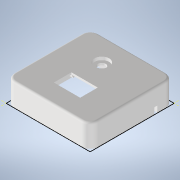
# Autodesk Inventor part: Deckel
Saved by Autodesk Inventor 2022.2 (Build 262287000, 287)
## iProperties
Created: 2022-01-23
Part Number: Deckel
Material: Generisch
Document SubType Name: Modeling
Designer: hpcwoess
Density: 1 g/cm^3
Appearance: Vorgabe
Author: hpcwoess
Autodesk Inventor part; units mm, degrees
ref_plane "YZ Plane" through (0, 0, 0) normal (1, 0, 0) x (0, 1, 0)
ref_plane "XZ Plane" through (0, 0, 0) normal (0, 1, 0) x (-1, 0, 0)
ref_plane "XY Plane" through (0, 0, 0) normal (0, 0, 1) x (1, 0, 0)
sketch "Skizze1" plane through (0, 0, 0) normal (0, 1, 0) x (-1, 0, 0)
  line L0 (30.3, 19.3) -> (-30.3, 19.3)
  line L1 (-30.3, 19.3) -> (-30.3, -34.9)
  line L2 (-30.3, -34.9) -> (30.3, -34.9)
  line L3 (30.3, -34.9) -> (30.3, 19.3)
  line L4 (40.5, -43.7) -> (-40.5, -43.7)
  line L5 (-40.5, -43.7) -> (-40.5, 37.3)
  line L6 (-40.5, 37.3) -> (40.5, 37.3)
  line L7 (40.5, 37.3) -> (40.5, -43.7)
  point P0 (0, 0)
  dimension "d0" = 30.3
  dimension "d1" = 60.6
  dimension "d2" = 54.2
  dimension "d3" = 19.3
  dimension "d4" = 81
  dimension "d5" = 81
  dimension "d6" = 40.5
  dimension "d7" = 18
  constraints: 16 end point, 4 parallel, 2 horizontal, 2 perpendicular
  measures "d0" distance from line of L3 point (0, 0)
  measures "d1" distance of L0.start L0.end
  measures "d2" distance of L2.end L0.start
  measures "d3" distance from line of L0 point (0, 0)
  measures "d4" distance of L5.end L6.end
  measures "d5" distance of L4.end L5.end
  measures "d6" distance from line of L5 point (0, 0)
  measures "d7" distance between parallel lines of L6 L0
extrude "Extrusion1" add sketch "Skizze1" along normal blind 20
sketch "Skizze2" plane through (0, 0, 0) normal (0, -1, 0) x (1, 0, 0)
  line L0 (-40.5, 37.3) -> (40.5, 37.3)
  line L1 (40.5, 37.3) -> (40.5, -43.7)
  line L2 (40.5, -43.7) -> (-40.5, -43.7)
  line L3 (-40.5, -43.7) -> (-40.5, 37.3)
  point P0 (0, 0)
  constraints: 8 end point, 2 parallel, 1 horizontal, 1 perpendicular
sketch "Skizze3" plane through (0, 20, 0) normal (0, 1, 0) x (1, 0, 0)
  line L0 (30.3, -19.3) -> (-30.3, -19.3) projected
  line L1 (25, -19.3) -> (-25, -19.3)
  line L2 (-25, -19.3) -> (-25, -31.3)
  line L3 (-25, -31.3) -> (25, -31.3)
  line L4 (25, -31.3) -> (25, -19.3)
  point P0 (0, 0)
  point P1 (-25, -19.3)
  dimension "d12" = 12
  dimension "d13" = 50
  dimension "d14" = 25
  constraints: 8 end point, 2 parallel, 1 horizontal, 1 perpendicular, 1 point on line
  measures "d12" distance of L3.end L1.start
  measures "d13" distance of L2.end L3.end
  measures "d14" distance from line of L4 point (0, 0)
extrude "Extrusion3" cut sketch "Skizze3" against normal blind 20
sketch "Skizze4" plane through (0, 20, 0) normal (0, 1, 0) x (1, 0, 0)
  line L0 (-40.5, -37.3) -> (40.5, -37.3) projected
  line L1 (-40.5, 43.7) -> (-40.5, -37.3) projected
  line L2 (40.5, -37.3) -> (-40.5, -37.3)
  line L3 (-40.5, -37.3) -> (-40.5, 43.7)
  line L4 (-40.5, 43.7) -> (40.5, 43.7)
  line L5 (40.5, 43.7) -> (40.5, -37.3)
  point P0 (0, 0)
  constraints: 8 end point, 2 parallel, 1 horizontal, 1 perpendicular
extrude "Extrusion4" add sketch "Skizze4" along normal blind 2
sketch "Skizze5" plane through (0, 20, 0) normal (0, -1, 0) x (1, 0, 0)
  line L0 (-12.7, 19) -> (12.7, 19)
  line L1 (12.7, 19) -> (12.7, 2)
  line L2 (12.7, 2) -> (-12.7, 2)
  line L3 (-12.7, 2) -> (-12.7, 19)
  point P0 (0, 0)
  dimension "d19" = 25.4
  dimension "d20" = 17
  dimension "d21" = 12.7
  dimension "d22" = 2
  constraints: 8 end point, 2 parallel, 1 horizontal, 1 perpendicular
  measures "d19" distance of L1.end L2.end
  measures "d20" distance of L0.end L1.end
  measures "d21" distance from line of point (0, 0) L1
  measures "d22" distance from line of L2 point (0, 0)
extrude "Extrusion5" cut sketch "Skizze5" against normal blind 20
sketch "Skizze6" plane through (0, 20, 0) normal (0, -1, 0) x (1, 0, 0)
  line L0 (-12.5757, 21) -> (12.5757, 21)
  line L1 (12.5757, 21) -> (12.5757, 23)
  line L2 (12.5757, 23) -> (-12.5757, 23)
  line L3 (-12.5757, 23) -> (-12.5757, 21)
  line L4 (-12.7, 19) -> (12.7, 19) projected
  point P0 (0, 0)
  dimension "d25" = 2
  dimension "d26" = 2
  constraints: 8 end point, 2 parallel, 1 horizontal, 1 perpendicular
  measures "d25" distance of L0.end L1.end
  measures "d26" distance between parallel lines of L4 L0
extrude "Extrusion6" cut sketch "Skizze6" against normal blind 1
sketch "Skizze7" plane through (0, 20, 0) normal (0, -1, 0) x (1, 0, 0)
  line L0 (-15.7, -3.5) -> (-11.7, -3.5)
  line L1 (-11.7, -3.5) -> (-11.7, 1.5)
  line L2 (-11.7, 1.5) -> (-15.7, 1.5)
  line L3 (-15.7, 1.5) -> (-15.7, -3.5)
  line L4 (-15.7, 19.5) -> (-11.7, 19.5)
  line L5 (-11.7, 19.5) -> (-11.7, 24.5)
  line L6 (-11.7, 24.5) -> (-15.7, 24.5)
  line L7 (-15.7, 24.5) -> (-15.7, 19.5)
  line L8 (12.7, 2) -> (-12.7, 2) projected
  line L9 (-12.7, 19) -> (12.7, 19) projected
  line L10 (-12.7, 2) -> (-12.7, 19) projected
  point P0 (0, 0)
  point P1 (-11.7, 22)
  dimension "d29" = 4
  dimension "d30" = 0.5
  dimension "d31" = 5
  dimension "d32" = 5
  dimension "d33" = 0.5
  dimension "d34" = 1
  constraints: 16 end point, 4 parallel, 2 horizontal, 2 perpendicular, 2 point on line, 1 midpoint
  measures "d29" distance of L0.start L0.end
  measures "d30" distance between parallel lines of L8 L2
  measures "d31" distance of L2.end L0.start
  measures "d32" distance of L4.end L5.end
  measures "d33" distance between parallel lines of L9 L4
  measures "d34" distance from line of L10 point (-11.7, 22)
extrude "Extrusion7" add sketch "Skizze7" along normal blind 2.5
sketch "Skizze8" plane through (-11.7, 20, -3.5) normal (0, 0, -1) x (-1, 0, 0)
  line L0 (0, 0) -> (0, -2.5) projected
  line L1 (0, 0) -> (1, 0)
  line L2 (1, 0) -> (1, -1.4)
  line L3 (1, -1.4) -> (0, -1.4)
  line L4 (0, -1.4) -> (0, 0)
  point P0 (-11.7, -20)
  point P1 (0, -1.4)
  dimension "d37" = 1
  dimension "d38" = 1.4
  constraints: 8 end point, 2 parallel, 1 horizontal, 1 perpendicular
  measures "d37" distance of L2.end L3.end
  measures "d38" distance of L1.end L2.end
extrude "Extrusion8" cut sketch "Skizze8" against normal blind 29.5
fillet "Rundung1" radius 8 4 edges at (40.5, 11, 37.3) (40.5, 11, -43.7) (-40.5, 11, 37.3) (-40.5, 11, -43.7)
fillet "Rundung2" radius 2 8 edges at (38.1569, 22, -41.3569) (0, 22, -43.7) (-38.1569, 22, -41.3569) (-40.5, 22, -3.2) (-38.1569, 22, 34.9569) (0, 22, 37.3) (38.1569, 22, 34.9569) (40.5, 22, -3.2)
sketch "Skizze9" plane through (-30.3, 0, 19.3) normal (1, 0, 0) x (0, 0, -1)
  line L0 (54, 11) -> (57, 0)
  line L1 (63, 0) -> (55, 0) projected
  line L2 (57, 0) -> (54, 0)
  line L3 (54, 0) -> (54, 11)
  line L4 (53.8, 6) -> (53.8, 11) projected
  line L5 (53.8, 6) -> (53.8, 2) projected
  line L6 (49.8, 6) -> (53.8, 6) projected
  line L7 (49.8, 2) -> (49.8, 6) projected
  line L8 (49.8, 2) -> (53.8, 2) projected
  line L9 (49.8, 6) -> (53.8, 6) projected
  line L10 (53.8, 6) -> (53.8, 11) projected
  line L11 (49.8, 11) -> (53.8, 11) projected
  line L12 (49.8, 8.9) -> (49.8, 11) projected
  line L13 (49.8, 8.9) -> (51.8, 8.9) projected
  line L14 (51.8, 8.9) -> (51.8, 7) projected
  line L15 (51.8, 7) -> (49.8, 7) projected
  line L16 (49.8, 6) -> (49.8, 7) projected
  point P0 (19.3, 0)
  dimension "d45" = 11
  dimension "d46" = 9
  dimension "d47" = 3
  constraints: 6 end point, 1 horizontal, 1 perpendicular, 1 point on line
  measures "d45" distance of L2.end L0.start
  measures "d46" distance from line of L1.start L3
  measures "d47" distance of L0.end L2.end
extrude "Extrusion9" cut sketch "Skizze9" along normal up to surface (60.6 mm away) contours L0 L1 L2 L3
sketch "Skizze10" plane through (-25, 0, 31.3) normal (1, 0, 0) x (0, 0, -1)
  line L0 (16.3, 6) -> (12.3, 6) projected
  line L1 (12.3, 2) -> (31.3, 2) projected
  line L2 (12, 0) -> (12, 20) projected
  arc A0 (12, 2) -> (12, 6) centre (11.4824, 4) ccw
  line L3 (12, 2) -> (12, 6)
  point P0 (31.3, 0)
  constraints: 3 point on line, 2 end point, 2 point on circle, 1 centre point, 1 collinear
extrude "Extrusion10" add sketch "Skizze10" against normal blind 10
sketch "Skizze11" plane through (25, 0, 19.3) normal (-1, 0, 0) x (0, 0, 1)
  line L0 (12, 20) -> (0, 20) projected
  line L1 (12, 20) -> (12, 0) projected
  line L2 (0, 0) -> (12, 0) projected
  line L3 (0, 2) -> (0, 0) projected
  arc A0 (0, 6) -> (0, 2) centre (0.5176, 4) ccw projected
  line L4 (0, 20) -> (0, 6) projected
  line L5 (0, 6) -> (0, 2)
  line L6 (0, 0) -> (0, 20) projected
  arc A1 (0, 2) -> (0, 2) centre (0.512, 3.9787) ccw
  point P0 (-19.3, 0)
  constraints: 3 point on circle, 2 end point, 1 centre point, 1 collinear, 1 tangent
extrude "Extrusion11" add sketch "Skizze11" against normal blind 10 contours A0 L5 A1 | A1 L5 picked at (-0.1516, 3.3785)
sketch "Skizze12" plane through (0, 20, 0) normal (0, -1, 0) x (1, 0, 0)
  circle A0 centre (-6.3, -20.9) radius 3.75
  line L0 (-30.3, -34.9) -> (30.3, -34.9) projected
  line L1 (-30.3, 19.3) -> (-30.3, -37.7) projected
  point P0 (0, 0)
  dimension "d52" = 14
  dimension "d53" = 24
  dimension "d54" = 7.5
  constraints: 1 centre point
  measures "d52" distance from line of A0.centre L0
  measures "d53" distance from line of A0.centre L1
  measures "d54" diameter of A0
extrude "Extrusion12" cut sketch "Skizze12" against normal blind 10
sketch "Skizze13" plane through (0, 20, 0) normal (0, -1, 0) x (1, 0, 0)
  circle A0 centre (-6.3, -20.9) radius 4.75
  circle A1 centre (-6.3, -20.9) radius 9
  point P0 (0, 0)
  dimension "d57" = 18
  dimension "d70" = 9.5
  constraints: 2 centre point, 1 coincident
  measures "d57" diameter of A1
  measures "d70" diameter of A0
extrude "Extrusion13" add sketch "Skizze13" along normal blind 3 contours A0 | A1
sketch "Skizze14" plane through (-6.3, 20, -20.9) normal (0, 1, 0) x (1, 0, 0)
  circle A0 centre (0, 0) radius 3.75 projected
  point P0 (6.3, -20.9)
extrude "Extrusion14" cut sketch "Skizze14" against normal through all
sketch "Skizze15" plane through (0, 22, 0) normal (0, 1, 0) x (1, 0, 0)
  circle A0 centre (-6.3, 20.9) radius 3.75 projected
  circle A1 centre (-6.3, 20.9) radius 7
  point P0 (0, 0)
  dimension "d62" = 14
  constraints: 1 centre point, 1 coincident
  measures "d62" diameter of A1
extrude "Extrusion15" cut sketch "Skizze15" against normal blind 3
sketch "Skizze16" plane through (40.5, 0, 29.3) normal (1, 0, 0) x (0, 0, -1)
  line L0 (67, 0) -> (10, 0) projected
  line L1 (54, 0) -> (57, 0)
  line L2 (57, 0) -> (57, 6)
  line L3 (57, 6) -> (54, 6)
  line L4 (54, 6) -> (54, 0)
  line L5 (73, 0) -> (73, 20) projected
  point P0 (29.3, 0)
  dimension "d65" = 6
  dimension "d66" = 3
  dimension "d67" = 16
  constraints: 8 end point, 2 parallel, 1 horizontal, 1 perpendicular, 1 point on line
  measures "d65" distance of L3.end L1.start
  measures "d66" distance of L2.end L3.end
  measures "d67" distance between parallel lines of L5 L2
extrude "Extrusion16" cut sketch "Skizze16" against normal blind 27.75
equation "\"d0\" = 0.5 * d1"
equation "\"d6\" = 0.5 * d4"
equation "\"d14\" = 0.5 * d13"
equation "\"d21\" = 0.5 * d19"
